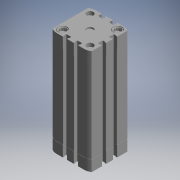
# Autodesk Inventor part: 536288 ADN-100-P---(Z)
Saved by Autodesk Inventor 2017.3 (Build 213256000, 256)
## iProperties
Part Number: 536288 ADN-100-P---(Z)
Material: Generic
Catalog Web Link: www.cadenas.de
Description: ADN-(Z)-Compact cylinder - Z
Vendor: FESTO
Document SubType Name: Modeling
Designer: partserver
Manufacturer: FESTO
Mass: 233.026 g
Surface Area: 768.338 cm^2
Volume: 233.026 cm^3
Density: 1 g/cm^3
Appearance: PSOLRGB-191-191-191
Category: PARTsolutions
Company: FESTO
Title: 536288 ADN-100-P---(Z)
Author: Cadenas PARTsolutions
Comments: Compact cylinder - Z
PSOL_IDENT_0: {$CADENAS_DATA\23d-libs\festo\parts\a\adn\parts\adn_zr.prj},213 {VTYP=3D},{NB=536288 ADN-100-P---(Z)
PSOL_IDENT_1: },{LINA=536288 ADN-100-P---(Z)},{NN=ADN-(Z)},{DATE=20.11.2019 12:35:12},{GEOMDATE=10.12.2018 13:24:4
PSOL_IDENT_2: 7},{VERSION=},{LINEID=8210},{WBVAR=HUB,DF,Q,S2S20,S1,R8,TT},{WBNUMERIC=HUB}  {NB=536288 ADN-100-P---
PSOL_IDENT_3: (Z)},{LINA=536288 ADN-100-P---(Z)},{KT=536288},{TNR=536288},{AUSF=ADN},{KDM=40},{BG=26.000},{VERS=2}
PSOL_IDENT_4: ,{HUBP=-},{HUB=100.00000},{HUB1=[1-400]},{HUB2=[1-300]},{HUB3=[10-400]},{THC='A','I'},{DF=P},{GA=A},
PSOL_IDENT_5: {HUBL=variable},{HUBC=hubc error},{Q=-},{VAR1C='-','Q'},{S2S20=-},{VAR2C='-','S2','S20'},{VAR5C='-','
PSOL_IDENT_6: S6'},{S1=-},{R8=-},{R81='-','R8'},{TT=-},{TT1='-','TT'},{VAR6C='-','S1'},{VAR7C='-','R3'},{HUBALG=[1
PSOL_IDENT_7: -400]},{A=19.000},{A1=22.000},{AF=16.000},{AF1=0.000},{AF2=14.000},{AF3=20.000},{B=35.000},{B1=27.00
PSOL_IDENT_8: 0},{BG1=16.000},{D1=9.000},{D2=9.000},{D3=5.100},{D4=17.000},{D5=8.000},{D6=M5},{D7=5.000},{D8=4.500
PSOL_IDENT_9: },{D9=8.000},{E=54.500},{EE=G1/8},{EEN=9.728},{EE1=M5},{J=15.000},{J1=8.000},{J11=8},{J2=15.000},{KF=
PSOL_IDENT_10: 5/16-24 UNF-2B},{KF1=-},{KF2=10-32 UNF-2B},{KF3=3/8-24 UNF-2B},{KK=3/8-24 UNF-2A},{KK1=1/2-20 UNF-2A
PSOL_IDENT_11: },{L1=3.300},{L2=45.000},{L3=2.100},{L4=5.000},{L5=6.000},{L6=61.000},{L7=33.000},{L8=3.000},{L9=2.6
PSOL_IDENT_12: 00},{L10=5.000},{L11=4.700},{MF=10.000},{MM=12.000},{MM1=16.000},{PL=8.200},{RT=M6},{RTN=6},{RTNK=4.
PSOL_IDENT_13: 917},{SF=3/8},{SF1=1/2},{SW=10.000},{TG=38.000},{VD=9.500},{VD1=6.400},{WH=6.200},{WH1=17.750},{WL=4
PSOL_IDENT_14: .700},{WL1=6.500},{Y1=0.400},{Y2=0.600},{ZJ=51.200},{ZM=57.400},{RU=43.600},{R1=14.800},{R2=1.000},{
PSOL_IDENT_15: RA=15.200},{RB1=5.400},{RB2=6.800},{RT1=3.400},{DSK=9.000},{MDK=13.000},{MK=8.000},{MT=4.000},{MS=6.
PSOL_IDENT_16: 000},{RUB=0.600},{KFN=8.000},{KFK=6.647},{B111=12.800},{B11=1.000},{B2=7.000},{B3=11.900},{B4=4.600}
PSOL_IDENT_17: ,{B5=4.400},{B6=8.500},{B7=26.000},{B8=6.000},{B9=9.000},{B10=10.000},{W=0.400},{S=8.000},{LA=15.000
PSOL_IDENT_18: },{LA1=5.000},{LA2=8.000},{LA3=12.500},{LA31=12.500},{LA4=8.200},{LA5=5.000},{LA6=11.000},{RR=6.000}
PSOL_IDENT_19: ,{LA7=0.000},{LA8=0.000},{LA9=0.000},{LA10=0.000},{ES=0.000},{SS=0.000},{TS=0.000},{WS=0.000},{DK=0.
PSOL_IDENT_20: 000},{KS=0.000},{QN=},{S2N=},{S1S20N=},{R8N=},{TTN=},{DFALG='P','PPS'}
NB: 536288 ADN-100-P---(Z)
NN: ADN-(Z)
NT: Compact cylinder - Z
NBSYN: $TNR. $AUSF.-$HUB.-$DF.$QN.$S2N.$S1S20N.$R8N.$TTN.---(Z)
LINA: 536288 ADN-100-P---(Z)
CATALOG: Festo
TNR: 536288
AUSF: ADN
KDM: 40
BG: 26
HUB: 100
DF: P
GA: A
Q: -
S2S20: -
S1: -
R8: -
TT: -
A: 19
A1: 22
AF: 16
AF1: 0
AF2: 14
AF3: 20
B: 35
B1: 27
BG1: 16
D1: 9
D2: 9
D3: 5.1
D4: 17
D5: 8
D6: M5
D7: 5
D8: 4.5
D9: 8
E: 54.5
EE: G1/8
EE1: M5
J: 15
J1: 8
J2: 15
KF: 5/16-24 UNF-2B
KF1: -
KF2: 10-32 UNF-2B
KF3: 3/8-24 UNF-2B
KK: 3/8-24 UNF-2A
KK1: 1/2-20 UNF-2A
L1: 3.3
L2: 45
L3: 2.1
L4: 5
L5: 6
L6: 61
L7: 33
L8: 3
L9: 2.6
L10: 5
L11: 4.7
MF: 10
MM: 12
MM1: 16
PL: 8.2
RT: M6
RTNK: 4.917
SF: 3/8
SF1: 1/2
SW: 10
TG: 38
VD: 9.5
VD1: 6.4
WH: 6.2
WH1: 17.75
WL: 4.7
WL1: 6.5
Y1: 0.4
Y2: 0.6
ZJ: 51.2
ZM: 57.4
RU: 43.6
R1: 14.8
R2: 1
RA: 15.2
DSK: 9
MDK: 13
MK: 8
MT: 4
MS: 6
RUB: 0.6
B111: 12.8
B11: 1
B2: 7
B3: 11.9
B4: 4.6
B5: 4.4
B6: 8.5
B7: 26
B8: 6
B9: 9
B10: 10
W: 0.4
S: 8
LA: 15
LA1: 5
LA2: 8
LA3: 12.5
LA31: 12.5
LA4: 8.2
LA5: 5
LA6: 11
RR: 6
LA7: 0
LA8: 0
LA9: 0
LA10: 0
ES: 0
SS: 0
TS: 0
WS: 0
DK: 0
KS: 0
SUPPLIER: FESTO
ARTICLENO: 536288 ADN-100-P---(Z)
BOMINFO: 536288 ADN-100-P---(Z)
CREATOR: CADENAS GmbH
Autodesk Inventor part; units mm, degrees
sketch "Skizze_2" plane through (0, 0, 0) normal (0, 0, 1) x (1, 0, 0)
  arc A0 (-27.25, -4.5) -> (-26.85, -4.9) centre (-26.85, -4.5) ccw
  line L0 (-26.85, -4.9) -> (-25.4, -4.9)
  arc A1 (-25.4, -4.9) -> (-25.2, -4.7) centre (-25.4, -4.7) ccw
  line L1 (-25.2, -4.7) -> (-25.2, -4.4)
  arc A2 (-25, -4.2) -> (-25.2, -4.4) centre (-25, -4.4) ccw
  line L2 (-25, -4.2) -> (-22.2, -4.2)
  arc A3 (-21.8, -4.6) -> (-22.2, -4.2) centre (-22.2, -4.6) ccw
  line L3 (-21.8, -4.6) -> (-21.8, -10.6)
  arc A4 (-22.2, -11) -> (-21.8, -10.6) centre (-22.2, -10.6) ccw
  line L4 (-22.2, -11) -> (-25, -11)
  arc A5 (-25.2, -10.8) -> (-25, -11) centre (-25, -10.8) ccw
  line L5 (-25.2, -10.8) -> (-25.2, -10.5)
  arc A6 (-25.2, -10.5) -> (-25.4, -10.3) centre (-25.4, -10.5) ccw
  line L6 (-25.4, -10.3) -> (-26.85, -10.3)
  arc A7 (-26.85, -10.3) -> (-27.25, -10.7) centre (-26.85, -10.7) ccw
  line L7 (-27.25, -10.7) -> (-27.25, -24.1921)
  arc A8 (-27.25, -24.1921) -> (-26.7754, -25.043) centre (-26.25, -24.1921) ccw
  arc A9 (-26.7754, -25.043) -> (-19, -27.25) centre (-19, -12.45) ccw
  line L8 (-19, -27.25) -> (-10.7, -27.25)
  arc A10 (-10.7, -27.25) -> (-10.3, -26.85) centre (-10.7, -26.85) ccw
  line L9 (-10.3, -26.85) -> (-10.3, -25.4)
  arc A11 (-10.3, -25.4) -> (-10.5, -25.2) centre (-10.5, -25.4) ccw
  line L10 (-10.5, -25.2) -> (-10.8, -25.2)
  arc A12 (-11, -25) -> (-10.8, -25.2) centre (-10.8, -25) ccw
  line L11 (-11, -25) -> (-11, -22.2)
  arc A13 (-10.6, -21.8) -> (-11, -22.2) centre (-10.6, -22.2) ccw
  line L12 (-10.6, -21.8) -> (-4.6, -21.8)
  arc A14 (-4.2, -22.2) -> (-4.6, -21.8) centre (-4.6, -22.2) ccw
  line L13 (-4.2, -22.2) -> (-4.2, -25)
  arc A15 (-4.4, -25.2) -> (-4.2, -25) centre (-4.4, -25) ccw
  line L14 (-4.4, -25.2) -> (-4.7, -25.2)
  arc A16 (-4.7, -25.2) -> (-4.9, -25.4) centre (-4.7, -25.4) ccw
  line L15 (-4.9, -25.4) -> (-4.9, -26.85)
  arc A17 (-4.9, -26.85) -> (-4.5, -27.25) centre (-4.5, -26.85) ccw
  line L16 (-4.5, -27.25) -> (4.5, -27.25)
  arc A18 (4.5, -27.25) -> (4.9, -26.85) centre (4.5, -26.85) ccw
  line L17 (4.9, -26.85) -> (4.9, -25.4)
  arc A19 (4.9, -25.4) -> (4.7, -25.2) centre (4.7, -25.4) ccw
  line L18 (4.7, -25.2) -> (4.4, -25.2)
  arc A20 (4.2, -25) -> (4.4, -25.2) centre (4.4, -25) ccw
  line L19 (4.2, -25) -> (4.2, -22.2)
  arc A21 (4.6, -21.8) -> (4.2, -22.2) centre (4.6, -22.2) ccw
  line L20 (4.6, -21.8) -> (10.6, -21.8)
  arc A22 (11, -22.2) -> (10.6, -21.8) centre (10.6, -22.2) ccw
  line L21 (11, -22.2) -> (11, -25)
  arc A23 (10.8, -25.2) -> (11, -25) centre (10.8, -25) ccw
  line L22 (10.8, -25.2) -> (10.5, -25.2)
  arc A24 (10.5, -25.2) -> (10.3, -25.4) centre (10.5, -25.4) ccw
  line L23 (10.3, -25.4) -> (10.3, -26.85)
  arc A25 (10.3, -26.85) -> (10.7, -27.25) centre (10.7, -26.85) ccw
  line L24 (10.7, -27.25) -> (19, -27.25)
  arc A26 (19, -27.25) -> (26.7754, -25.043) centre (19, -12.45) ccw
  arc A27 (26.7754, -25.043) -> (27.25, -24.1921) centre (26.25, -24.1921) ccw
  line L25 (27.25, -24.1921) -> (27.25, 24.1921)
  arc A28 (27.25, 24.1921) -> (26.7754, 25.043) centre (26.25, 24.1921) ccw
  arc A29 (26.7754, 25.043) -> (19, 27.25) centre (19, 12.45) ccw
  line L26 (19, 27.25) -> (10.7, 27.25)
  arc A30 (10.7, 27.25) -> (10.3, 26.85) centre (10.7, 26.85) ccw
  line L27 (10.3, 26.85) -> (10.3, 25.4)
  arc A31 (10.3, 25.4) -> (10.5, 25.2) centre (10.5, 25.4) ccw
  line L28 (10.5, 25.2) -> (10.8, 25.2)
  arc A32 (11, 25) -> (10.8, 25.2) centre (10.8, 25) ccw
  line L29 (11, 25) -> (11, 22.2)
  arc A33 (10.6, 21.8) -> (11, 22.2) centre (10.6, 22.2) ccw
  line L30 (10.6, 21.8) -> (4.6, 21.8)
  arc A34 (4.2, 22.2) -> (4.6, 21.8) centre (4.6, 22.2) ccw
  line L31 (4.2, 22.2) -> (4.2, 25)
  arc A35 (4.4, 25.2) -> (4.2, 25) centre (4.4, 25) ccw
  line L32 (4.4, 25.2) -> (4.7, 25.2)
  arc A36 (4.7, 25.2) -> (4.9, 25.4) centre (4.7, 25.4) ccw
  line L33 (4.9, 25.4) -> (4.9, 26.85)
  arc A37 (4.9, 26.85) -> (4.5, 27.25) centre (4.5, 26.85) ccw
  line L34 (4.5, 27.25) -> (-4.5, 27.25)
  arc A38 (-4.5, 27.25) -> (-4.9, 26.85) centre (-4.5, 26.85) ccw
  line L35 (-4.9, 26.85) -> (-4.9, 25.4)
  arc A39 (-4.9, 25.4) -> (-4.7, 25.2) centre (-4.7, 25.4) ccw
  line L36 (-4.7, 25.2) -> (-4.4, 25.2)
  arc A40 (-4.2, 25) -> (-4.4, 25.2) centre (-4.4, 25) ccw
  line L37 (-4.2, 25) -> (-4.2, 22.2)
  arc A41 (-4.6, 21.8) -> (-4.2, 22.2) centre (-4.6, 22.2) ccw
  line L38 (-4.6, 21.8) -> (-10.6, 21.8)
  arc A42 (-11, 22.2) -> (-10.6, 21.8) centre (-10.6, 22.2) ccw
  line L39 (-11, 22.2) -> (-11, 25)
  arc A43 (-10.8, 25.2) -> (-11, 25) centre (-10.8, 25) ccw
  line L40 (-10.8, 25.2) -> (-10.5, 25.2)
  arc A44 (-10.5, 25.2) -> (-10.3, 25.4) centre (-10.5, 25.4) ccw
  line L41 (-10.3, 25.4) -> (-10.3, 26.85)
  arc A45 (-10.3, 26.85) -> (-10.7, 27.25) centre (-10.7, 26.85) ccw
  line L42 (-10.7, 27.25) -> (-19, 27.25)
  arc A46 (-19, 27.25) -> (-26.7754, 25.043) centre (-19, 12.45) ccw
  arc A47 (-26.7754, 25.043) -> (-27.25, 24.1921) centre (-26.25, 24.1921) ccw
  line L43 (-27.25, 24.1921) -> (-27.25, 10.7)
  arc A48 (-27.25, 10.7) -> (-26.85, 10.3) centre (-26.85, 10.7) ccw
  line L44 (-26.85, 10.3) -> (-25.4, 10.3)
  arc A49 (-25.4, 10.3) -> (-25.2, 10.5) centre (-25.4, 10.5) ccw
  line L45 (-25.2, 10.5) -> (-25.2, 10.8)
  arc A50 (-25, 11) -> (-25.2, 10.8) centre (-25, 10.8) ccw
  line L46 (-25, 11) -> (-22.2, 11)
  arc A51 (-21.8, 10.6) -> (-22.2, 11) centre (-22.2, 10.6) ccw
  line L47 (-21.8, 10.6) -> (-21.8, 4.6)
  arc A52 (-22.2, 4.2) -> (-21.8, 4.6) centre (-22.2, 4.6) ccw
  line L48 (-22.2, 4.2) -> (-25, 4.2)
  arc A53 (-25.2, 4.4) -> (-25, 4.2) centre (-25, 4.4) ccw
  line L49 (-25.2, 4.4) -> (-25.2, 4.7)
  arc A54 (-25.2, 4.7) -> (-25.4, 4.9) centre (-25.4, 4.7) ccw
  line L50 (-25.4, 4.9) -> (-26.85, 4.9)
  arc A55 (-26.85, 4.9) -> (-27.25, 4.5) centre (-26.85, 4.5) ccw
  line L51 (-27.25, 4.5) -> (-27.25, -4.5)
  constraints: 112 point on circle, 104 end point, 56 centre point
extrude "Extrusion1" add sketch "Skizze_2" against normal blind 145
sketch "Sketch_113" plane through (0, 0, -15) normal (0, 0, 1) x (1, 0, 0)
  line L0 (-54.5, -54.5) -> (54.5, -54.5)
  line L1 (54.5, -54.5) -> (54.5, 54.5)
  line L2 (54.5, 54.5) -> (-54.5, 54.5)
  line L3 (-54.5, 54.5) -> (-54.5, -54.5)
  arc A0 (-27, -4.5) -> (-26.6, -4.9) centre (-26.6, -4.5) ccw
  line L4 (-26.6, -4.9) -> (-25.2, -4.9)
  line L5 (-25.2, -4.9) -> (-25.2, -10.3)
  line L6 (-25.2, -10.3) -> (-26.6, -10.3)
  arc A1 (-26.6, -10.3) -> (-27, -10.7) centre (-26.6, -10.7) ccw
  line L7 (-27, -10.7) -> (-27, -24.0929)
  arc A2 (-27, -24.0929) -> (-26.5072, -24.9547) centre (-26, -24.0929) ccw
  arc A3 (-26.5072, -24.9547) -> (-19, -27) centre (-19, -12.2) ccw
  line L8 (-19, -27) -> (-10.7, -27)
  arc A4 (-10.7, -27) -> (-10.3, -26.6) centre (-10.7, -26.6) ccw
  line L9 (-10.3, -26.6) -> (-10.3, -25.2)
  line L10 (-10.3, -25.2) -> (-4.9, -25.2)
  line L11 (-4.9, -25.2) -> (-4.9, -26.6)
  arc A5 (-4.9, -26.6) -> (-4.5, -27) centre (-4.5, -26.6) ccw
  line L12 (-4.5, -27) -> (4.5, -27)
  arc A6 (4.5, -27) -> (4.9, -26.6) centre (4.5, -26.6) ccw
  line L13 (4.9, -26.6) -> (4.9, -25.2)
  line L14 (4.9, -25.2) -> (10.3, -25.2)
  line L15 (10.3, -25.2) -> (10.3, -26.6)
  arc A7 (10.3, -26.6) -> (10.7, -27) centre (10.7, -26.6) ccw
  line L16 (10.7, -27) -> (19, -27)
  arc A8 (19, -27) -> (26.5072, -24.9547) centre (19, -12.2) ccw
  arc A9 (26.5072, -24.9547) -> (27, -24.0929) centre (26, -24.0929) ccw
  line L17 (27, -24.0929) -> (27, 24.0929)
  arc A10 (27, 24.0929) -> (26.5072, 24.9547) centre (26, 24.0929) ccw
  arc A11 (26.5072, 24.9547) -> (19, 27) centre (19, 12.2) ccw
  line L18 (19, 27) -> (10.7, 27)
  arc A12 (10.7, 27) -> (10.3, 26.6) centre (10.7, 26.6) ccw
  line L19 (10.3, 26.6) -> (10.3, 25.2)
  line L20 (10.3, 25.2) -> (4.9, 25.2)
  line L21 (4.9, 25.2) -> (4.9, 26.6)
  arc A13 (4.9, 26.6) -> (4.5, 27) centre (4.5, 26.6) ccw
  line L22 (4.5, 27) -> (-4.5, 27)
  arc A14 (-4.5, 27) -> (-4.9, 26.6) centre (-4.5, 26.6) ccw
  line L23 (-4.9, 26.6) -> (-4.9, 25.2)
  line L24 (-4.9, 25.2) -> (-10.3, 25.2)
  line L25 (-10.3, 25.2) -> (-10.3, 26.6)
  arc A15 (-10.3, 26.6) -> (-10.7, 27) centre (-10.7, 26.6) ccw
  line L26 (-10.7, 27) -> (-19, 27)
  arc A16 (-19, 27) -> (-26.5072, 24.9547) centre (-19, 12.2) ccw
  arc A17 (-26.5072, 24.9547) -> (-27, 24.0929) centre (-26, 24.0929) ccw
  line L27 (-27, 24.0929) -> (-27, 10.7)
  arc A18 (-27, 10.7) -> (-26.6, 10.3) centre (-26.6, 10.7) ccw
  line L28 (-26.6, 10.3) -> (-25.2, 10.3)
  line L29 (-25.2, 10.3) -> (-25.2, 4.9)
  line L30 (-25.2, 4.9) -> (-26.6, 4.9)
  arc A19 (-26.6, 4.9) -> (-27, 4.5) centre (-26.6, 4.5) ccw
  line L31 (-27, 4.5) -> (-27, -4.5)
  constraints: 64 end point, 40 point on circle, 20 centre point
extrude "Extrusion2" cut sketch "Sketch_113" against normal blind 115
sketch "Sketch3" plane through (27.25, -24.1921, 0) normal (1, 0, 0) x (0, 0, -1)
  point P0 (8.2, 16.1921)
hole "Hole1" at (27.25, -8, -8.2) direction (-1, 0, 0) diameter 8.566 depth 12.5 countersink diameter 9.728 countersink angle 90 thread size "G9.728x0.907" designation "G 1/8" standard "ISO Pipe Threads"
sketch "Sketch4" plane through (27.25, -24.1921, -145) normal (1, 0, 0) x (0, 0, -1)
  point P0 (-8.2, 32.1921)
hole "Hole2" at (27.25, 8, -136.8) direction (-1, 0, 0) diameter 8.566 depth 12.5 countersink diameter 9.728 countersink angle 90 thread size "G9.728x0.907" designation "G 1/8" standard "ISO Pipe Threads"
sketch "Skizze_5" plane through (0, 0, 0) normal (1, 0, 0) x (0, 1, 0)
  line L0 (0, -128.6) -> (0, 16.9)
  line L1 (0, 16.9) -> (6, 16.9)
  line L2 (6, 16.9) -> (6, -18.6)
  line L3 (6, -18.6) -> (20, -18.6)
  line L4 (20, -18.6) -> (20, -128.6)
  line L5 (20, -128.6) -> (0, -128.6)
  line L6 (0, -128.6) -> (0, 16.9)
  constraints: 14 end point
revolve "Revolution1" cut sketch "Skizze_5" angle 360 about axis through (0, 0, -128.6) along (0, 0, -1)
sketch "Sketch6" plane through (0, 0, -145) normal (0, 0, -1) x (-1, 0, 0)
  point P0 (0, 0)
hole "Hole3" at (0, 0, -145) direction (0, 0, 1) diameter 9 depth 2.1
sketch "Sketch7" plane through (0, 0, 0) normal (0, 0, 1) x (1, 0, 0)
  point P0 (19, 19)
hole "Hole4" at (19, 19, 0) direction (0, 0, -1) diameter 9 depth 26 counterbore diameter 12.8 counterbore depth 7
sketch "Sketch_27" plane through (19, 0, 0) normal (1, 0, 0) x (0, 0, -1)
  line L0 (26, 19) -> (0, 19)
  line L1 (0, 24) -> (1.299, 23.25)
  line L2 (1.299, 23.25) -> (4.6, 23.25)
  line L3 (4.6, 23.25) -> (4.6, 22)
  line L4 (4.6, 22) -> (5.1415, 21.4585)
  line L5 (5.1415, 21.4585) -> (26, 21.4585)
  line L6 (26, 21.4585) -> (26, 24.5)
  line L7 (26, 24.5) -> (7, 24.5)
  line L8 (7, 24.5) -> (7, 24.95)
  line L9 (7, 24.95) -> (0.4, 24.95)
  line L10 (0.4, 24.95) -> (0, 24.55)
  line L11 (0, 24.55) -> (0, 24)
  constraints: 24 end point
revolve "Revolution2" add sketch "Sketch_27" angle 360 about axis through (19, 19, -26) along (0, 0, -1)
thread "Thread1" size "M6x1" class "6H" standard "ISO Metric profile" full length
sketch "Sketch9" plane through (0, 0, -145) normal (0, 0, -1) x (-1, 0, 0)
  point P0 (-19, -19)
hole "Hole5" at (19, -19, -145) direction (0, 0, 1) diameter 9 depth 26 counterbore diameter 12.8 counterbore depth 7
sketch "Sketch_28" plane through (19, 0, 0) normal (1, 0, 0) x (0, 0, -1)
  line L0 (145, -19) -> (119, -19)
  line L1 (119, -13.5) -> (119, -16.5415)
  line L2 (119, -16.5415) -> (139.8585, -16.5415)
  line L3 (139.8585, -16.5415) -> (140.4, -16)
  line L4 (140.4, -16) -> (140.4, -14.75)
  line L5 (140.4, -14.75) -> (143.701, -14.75)
  line L6 (143.701, -14.75) -> (145, -14)
  line L7 (145, -14) -> (145, -13.45)
  line L8 (145, -13.45) -> (144.6, -13.05)
  line L9 (144.6, -13.05) -> (138, -13.05)
  line L10 (138, -13.05) -> (138, -13.5)
  line L11 (138, -13.5) -> (119, -13.5)
  constraints: 24 end point
revolve "Revolution3" add sketch "Sketch_28" angle 360 about axis through (19, -19, -145) along (0, 0, -1)
thread "Thread2" size "M6x1" class "6H" standard "ISO Metric profile" full length
sketch "Sketch11" plane through (0, 0, 0) normal (0, 0, 1) x (1, 0, 0)
  point P0 (-19, -19)
hole "Hole6" at (-19, -19, 0) direction (0, 0, -1) diameter 9 depth 26 counterbore diameter 12.8 counterbore depth 7
sketch "Sketch12" plane through (0, 0, -145) normal (0, 0, -1) x (-1, 0, 0)
  point P0 (19, 19)
hole "Hole7" at (-19, 19, -145) direction (0, 0, 1) diameter 9 depth 26 counterbore diameter 12.8 counterbore depth 7
sketch "Sketch_29" plane through (-19, 0, 0) normal (1, 0, 0) x (0, 0, -1)
  line L0 (26, -19) -> (0, -19)
  line L1 (0, -14) -> (1.299, -14.75)
  line L2 (1.299, -14.75) -> (4.6, -14.75)
  line L3 (4.6, -14.75) -> (4.6, -16)
  line L4 (4.6, -16) -> (5.1415, -16.5415)
  line L5 (5.1415, -16.5415) -> (26, -16.5415)
  line L6 (26, -16.5415) -> (26, -13.5)
  line L7 (26, -13.5) -> (7, -13.5)
  line L8 (7, -13.5) -> (7, -13.05)
  line L9 (7, -13.05) -> (0.4, -13.05)
  line L10 (0.4, -13.05) -> (0, -13.45)
  line L11 (0, -13.45) -> (0, -14)
  constraints: 24 end point
revolve "Revolution4" add sketch "Sketch_29" angle 360 about axis through (-19, -19, -26) along (0, 0, -1)
thread "Thread3" size "M6x1" class "6H" standard "ISO Metric profile" full length
sketch "Sketch_30" plane through (-19, 0, 0) normal (1, 0, 0) x (0, 0, -1)
  line L0 (145, 19) -> (119, 19)
  line L1 (119, 24.5) -> (119, 21.4585)
  line L2 (119, 21.4585) -> (139.8585, 21.4585)
  line L3 (139.8585, 21.4585) -> (140.4, 22)
  line L4 (140.4, 22) -> (140.4, 23.25)
  line L5 (140.4, 23.25) -> (143.701, 23.25)
  line L6 (143.701, 23.25) -> (145, 24)
  line L7 (145, 24) -> (145, 24.55)
  line L8 (145, 24.55) -> (144.6, 24.95)
  line L9 (144.6, 24.95) -> (138, 24.95)
  line L10 (138, 24.95) -> (138, 24.5)
  line L11 (138, 24.5) -> (119, 24.5)
  constraints: 24 end point
revolve "Revolution5" add sketch "Sketch_30" angle 360 about axis through (-19, 19, -145) along (0, 0, -1)
thread "Thread4" size "M6x1" class "6H" standard "ISO Metric profile" full length
sketch "Skizze_12" plane through (19, 0, 0) normal (1, 0, 0) x (0, 0, -1)
  line L0 (119, -19) -> (-0.1, -19)
  line L1 (-0.1, -19) -> (-0.1, -14.5)
  line L2 (-0.1, -14.5) -> (5, -14.5)
  line L3 (5, -14.5) -> (5, -16)
  line L4 (5, -16) -> (5.5415, -16.5415)
  line L5 (5.5415, -16.5415) -> (119, -16.5415)
  line L6 (119, -16.5415) -> (119, -19)
  line L7 (119, -19) -> (-0.1, -19)
  constraints: 16 end point
revolve "Revolution6" cut sketch "Skizze_12" angle 360 about axis through (19, -19, -119) along (0, 0, -1)
thread "Thread5" size "M6x1" class "6H" standard "ISO Metric profile" length 9.4585
sketch "Sketch_123" plane through (19, 0, 0) normal (1, 0, 0) x (0, 0, -1)
  line L0 (119, -19) -> (15, -19)
  line L1 (15, -19) -> (15, -14)
  line L2 (15, -14) -> (119, -14)
  line L3 (119, -14) -> (119, -19)
  line L4 (119, -19) -> (15, -19)
  constraints: 10 end point
revolve "Revolution7" add sketch "Sketch_123" angle 360 about axis through (19, -19, -119) along (0, 0, -1)
sketch "Sketch17" plane through (19, -19, -119) normal (0, 0, -1) x (-1, 0, 0)
  point P0 (0, 0)
hole "Hole8" at (19, -19, -119) direction (0, 0, 1) diameter 6 depth 104
sketch "Sketch_3" plane through (19, 0, 0) normal (1, 0, 0) x (0, 0, -1)
  line L0 (145.1, 19) -> (72.5, 19)
  line L1 (72.5, 19) -> (72.5, 21.4585)
  line L2 (72.5, 21.4585) -> (139.4585, 21.4585)
  line L3 (139.4585, 21.4585) -> (140, 22)
  line L4 (140, 22) -> (140, 23.5)
  line L5 (140, 23.5) -> (145.1, 23.5)
  line L6 (145.1, 23.5) -> (145.1, 19)
  line L7 (145.1, 19) -> (72.5, 19)
  constraints: 16 end point
revolve "Revolution8" cut sketch "Sketch_3" angle 360 about axis through (19, 19, -145.1) along (0, 0, -1)
thread "Thread6" size "M6x1" class "6H" standard "ISO Metric profile" length 9.4585
sketch "Sketch_117" plane through (19, 0, 0) normal (1, 0, 0) x (0, 0, -1)
  line L0 (130, 19) -> (26, 19)
  line L1 (26, 19) -> (26, 24)
  line L2 (26, 24) -> (130, 24)
  line L3 (130, 24) -> (130, 19)
  line L4 (130, 19) -> (26, 19)
  constraints: 10 end point
revolve "Revolution9" add sketch "Sketch_117" angle 360 about axis through (19, 19, -130) along (0, 0, -1)
sketch "Sketch20" plane through (19, 19, -130) normal (0, 0, -1) x (-1, 0, 0)
  point P0 (0, 0)
hole "Hole9" at (19, 19, -130) direction (0, 0, 1) diameter 6 depth 104
sketch "Skizze_13" plane through (-19, 0, 0) normal (1, 0, 0) x (0, 0, -1)
  line L0 (119, 19) -> (-0.1, 19)
  line L1 (-0.1, 19) -> (-0.1, 23.5)
  line L2 (-0.1, 23.5) -> (5, 23.5)
  line L3 (5, 23.5) -> (5, 22)
  line L4 (5, 22) -> (5.5415, 21.4585)
  line L5 (5.5415, 21.4585) -> (119, 21.4585)
  line L6 (119, 21.4585) -> (119, 19)
  line L7 (119, 19) -> (-0.1, 19)
  constraints: 16 end point
revolve "Revolution10" cut sketch "Skizze_13" angle 360 about axis through (-19, 19, -119) along (0, 0, -1)
thread "Thread7" size "M6x1" class "6H" standard "ISO Metric profile" length 9.4585
sketch "Sketch_121" plane through (-19, 0, 0) normal (1, 0, 0) x (0, 0, -1)
  line L0 (119, 19) -> (15, 19)
  line L1 (15, 19) -> (15, 24)
  line L2 (15, 24) -> (119, 24)
  line L3 (119, 24) -> (119, 19)
  line L4 (119, 19) -> (15, 19)
  constraints: 10 end point
revolve "Revolution11" add sketch "Sketch_121" angle 360 about axis through (-19, 19, -119) along (0, 0, -1)
sketch "Sketch23" plane through (-19, 19, -119) normal (0, 0, -1) x (-1, 0, 0)
  point P0 (0, 0)
hole "Hole10" at (-19, 19, -119) direction (0, 0, 1) diameter 6 depth 104
sketch "Sketch_4" plane through (-19, 0, 0) normal (1, 0, 0) x (0, 0, -1)
  line L0 (145.1, -19) -> (72.5, -19)
  line L1 (72.5, -19) -> (72.5, -16.5415)
  line L2 (72.5, -16.5415) -> (139.4585, -16.5415)
  line L3 (139.4585, -16.5415) -> (140, -16)
  line L4 (140, -16) -> (140, -14.5)
  line L5 (140, -14.5) -> (145.1, -14.5)
  line L6 (145.1, -14.5) -> (145.1, -19)
  line L7 (145.1, -19) -> (72.5, -19)
  constraints: 16 end point
revolve "Revolution12" cut sketch "Sketch_4" angle 360 about axis through (-19, -19, -145.1) along (0, 0, -1)
thread "Thread8" size "M6x1" class "6H" standard "ISO Metric profile" length 9.4585
sketch "Sketch_118" plane through (-19, 0, 0) normal (1, 0, 0) x (0, 0, -1)
  line L0 (130, -19) -> (26, -19)
  line L1 (26, -19) -> (26, -14)
  line L2 (26, -14) -> (130, -14)
  line L3 (130, -14) -> (130, -19)
  line L4 (130, -19) -> (26, -19)
  constraints: 10 end point
revolve "Revolution13" add sketch "Sketch_118" angle 360 about axis through (-19, -19, -130) along (0, 0, -1)
sketch "Sketch26" plane through (-19, -19, -130) normal (0, 0, -1) x (-1, 0, 0)
  point P0 (0, 0)
hole "Hole11" at (-19, -19, -130) direction (0, 0, 1) diameter 6 depth 104
sketch "Sketch_8" plane through (0, 0, 0) normal (0, 0, 1) x (1, 0, 0)
  line L0 (-23.6188, -19) -> (-23, -20.0718)
  line L1 (-23, -20.0718) -> (-23, -21.3094)
  line L2 (-23, -21.3094) -> (-21.9282, -21.9282)
  line L3 (-21.9282, -21.9282) -> (-21.3094, -23)
  line L4 (-21.3094, -23) -> (-20.0718, -23)
  line L5 (-20.0718, -23) -> (-19, -23.6188)
  line L6 (-19, -23.6188) -> (-17.9282, -23)
  line L7 (-17.9282, -23) -> (-16.6906, -23)
  line L8 (-16.6906, -23) -> (-16.0718, -21.9282)
  line L9 (-16.0718, -21.9282) -> (-15, -21.3094)
  line L10 (-15, -21.3094) -> (-15, -20.0718)
  line L11 (-15, -20.0718) -> (-14.3812, -19)
  line L12 (-14.3812, -19) -> (-15, -17.9282)
  line L13 (-15, -17.9282) -> (-15, -16.6906)
  line L14 (-15, -16.6906) -> (-16.0718, -16.0718)
  line L15 (-16.0718, -16.0718) -> (-16.6906, -15)
  line L16 (-16.6906, -15) -> (-17.9282, -15)
  line L17 (-17.9282, -15) -> (-19, -14.3812)
  line L18 (-19, -14.3812) -> (-20.0718, -15)
  line L19 (-20.0718, -15) -> (-21.3094, -15)
  line L20 (-21.3094, -15) -> (-21.9282, -16.0718)
  line L21 (-21.9282, -16.0718) -> (-23, -16.6906)
  line L22 (-23, -16.6906) -> (-23, -17.9282)
  line L23 (-23, -17.9282) -> (-23.6188, -19)
  constraints: 48 end point
extrude "Extrusion3" cut sketch "Sketch_8" against normal blind 4.4
sketch "Sketch_7" plane through (0, 0, 0) normal (0, 0, 1) x (1, 0, 0)
  line L0 (14.3812, 19) -> (15, 17.9282)
  line L1 (15, 17.9282) -> (15, 16.6906)
  line L2 (15, 16.6906) -> (16.0718, 16.0718)
  line L3 (16.0718, 16.0718) -> (16.6906, 15)
  line L4 (16.6906, 15) -> (17.9282, 15)
  line L5 (17.9282, 15) -> (19, 14.3812)
  line L6 (19, 14.3812) -> (20.0718, 15)
  line L7 (20.0718, 15) -> (21.3094, 15)
  line L8 (21.3094, 15) -> (21.9282, 16.0718)
  line L9 (21.9282, 16.0718) -> (23, 16.6906)
  line L10 (23, 16.6906) -> (23, 17.9282)
  line L11 (23, 17.9282) -> (23.6188, 19)
  line L12 (23.6188, 19) -> (23, 20.0718)
  line L13 (23, 20.0718) -> (23, 21.3094)
  line L14 (23, 21.3094) -> (21.9282, 21.9282)
  line L15 (21.9282, 21.9282) -> (21.3094, 23)
  line L16 (21.3094, 23) -> (20.0718, 23)
  line L17 (20.0718, 23) -> (19, 23.6188)
  line L18 (19, 23.6188) -> (17.9282, 23)
  line L19 (17.9282, 23) -> (16.6906, 23)
  line L20 (16.6906, 23) -> (16.0718, 21.9282)
  line L21 (16.0718, 21.9282) -> (15, 21.3094)
  line L22 (15, 21.3094) -> (15, 20.0718)
  line L23 (15, 20.0718) -> (14.3812, 19)
  constraints: 48 end point
extrude "Extrusion4" cut sketch "Sketch_7" against normal blind 4.4
sketch "Sketch_9" plane through (0, 0, -145) normal (0, 0, 1) x (1, 0, 0)
  line L0 (-23.6188, 19) -> (-23, 17.9282)
  line L1 (-23, 17.9282) -> (-23, 16.6906)
  line L2 (-23, 16.6906) -> (-21.9282, 16.0718)
  line L3 (-21.9282, 16.0718) -> (-21.3094, 15)
  line L4 (-21.3094, 15) -> (-20.0718, 15)
  line L5 (-20.0718, 15) -> (-19, 14.3812)
  line L6 (-19, 14.3812) -> (-17.9282, 15)
  line L7 (-17.9282, 15) -> (-16.6906, 15)
  line L8 (-16.6906, 15) -> (-16.0718, 16.0718)
  line L9 (-16.0718, 16.0718) -> (-15, 16.6906)
  line L10 (-15, 16.6906) -> (-15, 17.9282)
  line L11 (-15, 17.9282) -> (-14.3812, 19)
  line L12 (-14.3812, 19) -> (-15, 20.0718)
  line L13 (-15, 20.0718) -> (-15, 21.3094)
  line L14 (-15, 21.3094) -> (-16.0718, 21.9282)
  line L15 (-16.0718, 21.9282) -> (-16.6906, 23)
  line L16 (-16.6906, 23) -> (-17.9282, 23)
  line L17 (-17.9282, 23) -> (-19, 23.6188)
  line L18 (-19, 23.6188) -> (-20.0718, 23)
  line L19 (-20.0718, 23) -> (-21.3094, 23)
  line L20 (-21.3094, 23) -> (-21.9282, 21.9282)
  line L21 (-21.9282, 21.9282) -> (-23, 21.3094)
  line L22 (-23, 21.3094) -> (-23, 20.0718)
  line L23 (-23, 20.0718) -> (-23.6188, 19)
  constraints: 48 end point
extrude "Extrusion5" cut sketch "Sketch_9" along normal blind 4.4
sketch "Sketch_10" plane through (0, 0, -145) normal (0, 0, 1) x (1, 0, 0)
  line L0 (14.3812, -19) -> (15, -20.0718)
  line L1 (15, -20.0718) -> (15, -21.3094)
  line L2 (15, -21.3094) -> (16.0718, -21.9282)
  line L3 (16.0718, -21.9282) -> (16.6906, -23)
  line L4 (16.6906, -23) -> (17.9282, -23)
  line L5 (17.9282, -23) -> (19, -23.6188)
  line L6 (19, -23.6188) -> (20.0718, -23)
  line L7 (20.0718, -23) -> (21.3094, -23)
  line L8 (21.3094, -23) -> (21.9282, -21.9282)
  line L9 (21.9282, -21.9282) -> (23, -21.3094)
  line L10 (23, -21.3094) -> (23, -20.0718)
  line L11 (23, -20.0718) -> (23.6188, -19)
  line L12 (23.6188, -19) -> (23, -17.9282)
  line L13 (23, -17.9282) -> (23, -16.6906)
  line L14 (23, -16.6906) -> (21.9282, -16.0718)
  line L15 (21.9282, -16.0718) -> (21.3094, -15)
  line L16 (21.3094, -15) -> (20.0718, -15)
  line L17 (20.0718, -15) -> (19, -14.3812)
  line L18 (19, -14.3812) -> (17.9282, -15)
  line L19 (17.9282, -15) -> (16.6906, -15)
  line L20 (16.6906, -15) -> (16.0718, -16.0718)
  line L21 (16.0718, -16.0718) -> (15, -16.6906)
  line L22 (15, -16.6906) -> (15, -17.9282)
  line L23 (15, -17.9282) -> (14.3812, -19)
  constraints: 48 end point
extrude "Extrusion6" cut sketch "Sketch_10" along normal blind 4.4
ref_plane "CYLINDER_XY" through (0, 0, -128.6) normal (0, 0, 1) x (1, 0, 0)
ref_plane "CYLINDER_YZ" through (0, 0, -128.6) normal (1, 0, 0) x (0, 1, 0)
ref_plane "CYLINDER_ZX" through (0, 0, -128.6) normal (0, 1, 0) x (0, 0, 1)
ref_plane "FDT_FRONT_XY" through (0, 0, 0) normal (0, 0, 1) x (0, -1, 0)
ref_plane "FDT_FRONT_YZ" through (0, 0, 0) normal (0, -1, 0) x (1, 0, 0)
ref_plane "FDT_FRONT_ZX" through (0, 0, 0) normal (1, 0, 0) x (0, 0, 1)
ref_plane "FDT_QSFRONT_XY" through (27.25, -8, -8.2) normal (1, 0, 0) x (0, -1, 0)
ref_plane "FDT_QSFRONT_YZ" through (27.25, -8, -8.2) normal (0, -1, 0) x (0, 0, -1)
ref_plane "FDT_QSFRONT_ZX" through (27.25, -8, -8.2) normal (0, 0, -1) x (1, 0, 0)
ref_plane "FDT_QSREAR_XY" through (27.25, 8, -136.8) normal (1, 0, 0) x (0, -1, 0)
ref_plane "FDT_QSREAR_YZ" through (27.25, 8, -136.8) normal (0, -1, 0) x (0, 0, -1)
ref_plane "FDT_QSREAR_ZX" through (27.25, 8, -136.8) normal (0, 0, -1) x (1, 0, 0)
ref_plane "FDT_REAR_XY" through (0, 0, -145) normal (0, 0, 1) x (0, -1, 0)
ref_plane "FDT_REAR_YZ" through (0, 0, -145) normal (0, -1, 0) x (1, 0, 0)
ref_plane "FDT_REAR_ZX" through (0, 0, -145) normal (1, 0, 0) x (0, 0, 1)
ref_plane "FDT_SLOT3_XY" through (7.6, 21.8, -72.5) normal (0, 1, 0) x (1, 0, 0)
ref_plane "FDT_SLOT3_YZ" through (7.6, 21.8, -72.5) normal (1, 0, 0) x (0, 0, -1)
ref_plane "FDT_SLOT3_ZX" through (7.6, 21.8, -72.5) normal (0, 0, -1) x (0, 1, 0)
ref_plane "FDT_SLOT4_XY" through (-7.6, 21.8, -72.5) normal (0, 1, 0) x (1, 0, 0)
ref_plane "FDT_SLOT4_YZ" through (-7.6, 21.8, -72.5) normal (1, 0, 0) x (0, 0, -1)
ref_plane "FDT_SLOT4_ZX" through (-7.6, 21.8, -72.5) normal (0, 0, -1) x (0, 1, 0)
ref_plane "FDT_SLOT5_XY" through (-21.8, 7.6, -72.5) normal (-1, 0, 0) x (0, 1, 0)
ref_plane "FDT_SLOT5_YZ" through (-21.8, 7.6, -72.5) normal (0, 1, 0) x (0, 0, -1)
ref_plane "FDT_SLOT5_ZX" through (-21.8, 7.6, -72.5) normal (0, 0, -1) x (-1, 0, 0)
ref_plane "FDT_SLOT6_XY" through (-21.8, -7.6, -72.5) normal (-1, 0, 0) x (0, 1, 0)
ref_plane "FDT_SLOT6_YZ" through (-21.8, -7.6, -72.5) normal (0, 1, 0) x (0, 0, -1)
ref_plane "FDT_SLOT6_ZX" through (-21.8, -7.6, -72.5) normal (0, 0, -1) x (-1, 0, 0)
ref_plane "FDT_SLOT7_XY" through (-7.6, -21.8, -72.5) normal (0, -1, 0) x (-1, 0, 0)
ref_plane "FDT_SLOT7_YZ" through (-7.6, -21.8, -72.5) normal (-1, 0, 0) x (0, 0, -1)
ref_plane "FDT_SLOT7_ZX" through (-7.6, -21.8, -72.5) normal (0, 0, -1) x (0, -1, 0)
ref_plane "FDT_SLOT8_XY" through (7.6, -21.8, -72.5) normal (0, -1, 0) x (-1, 0, 0)
ref_plane "FDT_SLOT8_YZ" through (7.6, -21.8, -72.5) normal (-1, 0, 0) x (0, 0, -1)
ref_plane "FDT_SLOT8_ZX" through (7.6, -21.8, -72.5) normal (0, 0, -1) x (0, -1, 0)
ref_plane "TO_DUMMY_XY" through (0, 0, 0) normal (0, 0, 1) x (1, 0, 0)
ref_plane "TO_DUMMY_YZ" through (0, 0, 0) normal (1, 0, 0) x (0, 1, 0)
ref_plane "TO_DUMMY_ZX" through (0, 0, 0) normal (0, 1, 0) x (0, 0, 1)
body "Solid1"
